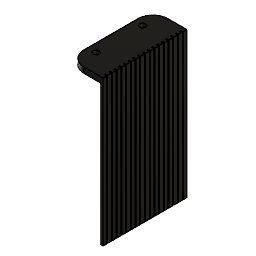
Cortina Lamas TPU (Autodesk Fusion 360 design; units mm, degrees)
Autodesk Fusion 360 part; units mm, degrees
note: some values were not read from the file. Set by a fixed rule: which sketch regions a step uses.
sketch "Boceto1" plane through (0, 0, 0) normal (0, 0, 1) x (1, 0, 0)
  circle A0 centre (0, 0) radius 1.575
  line L0 (0, 0) -> (12.5, 0)
  line L1 (12.5, 0) -> (12.5, 10)
  line L2 (12.5, 0) -> (12.5, -25)
  line L3 (12.5, 10) -> (-4.5, 10)
  line L4 (-4.5, 10) -> (-4.5, -35)
  line L5 (-4.5, -35) -> (12.5, -35)
  line L6 (12.5, -35) -> (12.5, 10)
  line L7 (12.5, -25) -> (0, -25)
  circle A1 centre (0, -25) radius 1.575
  line L8 (12.5, 10) -> (13.7, 10)
  line L9 (13.7, 10) -> (13.7, 8)
  line L10 (13.7, 8) -> (12.5, 8)
  line L11 (12.5, 8) -> (12.5, 10)
  line L12 (13.7, 5.4706) -> (12.5, 5.4706)
  line L13 (13.7, 7.4706) -> (13.7, 5.4706)
  line L14 (12.5, 7.4706) -> (13.7, 7.4706)
  line L15 (12.5, 5.4706) -> (12.5, 7.4706)
  line L16 (13.7, 2.9412) -> (12.5, 2.9412)
  line L17 (13.7, 4.9412) -> (13.7, 2.9412)
  line L18 (12.5, 4.9412) -> (13.7, 4.9412)
  line L19 (12.5, 2.9412) -> (12.5, 4.9412)
  line L20 (13.7, 0.4118) -> (12.5, 0.4118)
  line L21 (13.7, 2.4118) -> (13.7, 0.4118)
  line L22 (12.5, 2.4118) -> (13.7, 2.4118)
  line L23 (12.5, 0.4118) -> (12.5, 2.4118)
  line L24 (13.7, -2.1176) -> (12.5, -2.1176)
  line L25 (13.7, -0.1176) -> (13.7, -2.1176)
  line L26 (12.5, -0.1176) -> (13.7, -0.1176)
  line L27 (12.5, -2.1176) -> (12.5, -0.1176)
  line L28 (13.7, -4.6471) -> (12.5, -4.6471)
  line L29 (13.7, -2.6471) -> (13.7, -4.6471)
  line L30 (12.5, -2.6471) -> (13.7, -2.6471)
  line L31 (12.5, -4.6471) -> (12.5, -2.6471)
  line L32 (13.7, -7.1765) -> (12.5, -7.1765)
  line L33 (13.7, -5.1765) -> (13.7, -7.1765)
  line L34 (12.5, -5.1765) -> (13.7, -5.1765)
  line L35 (12.5, -7.1765) -> (12.5, -5.1765)
  line L36 (13.7, -9.7059) -> (12.5, -9.7059)
  line L37 (13.7, -7.7059) -> (13.7, -9.7059)
  line L38 (12.5, -7.7059) -> (13.7, -7.7059)
  line L39 (12.5, -9.7059) -> (12.5, -7.7059)
  line L40 (13.7, -12.2353) -> (12.5, -12.2353)
  line L41 (13.7, -10.2353) -> (13.7, -12.2353)
  line L42 (12.5, -10.2353) -> (13.7, -10.2353)
  line L43 (12.5, -12.2353) -> (12.5, -10.2353)
  line L44 (13.7, -14.7647) -> (12.5, -14.7647)
  line L45 (13.7, -12.7647) -> (13.7, -14.7647)
  line L46 (12.5, -12.7647) -> (13.7, -12.7647)
  line L47 (12.5, -14.7647) -> (12.5, -12.7647)
  line L48 (13.7, -17.2941) -> (12.5, -17.2941)
  line L49 (13.7, -15.2941) -> (13.7, -17.2941)
  line L50 (12.5, -15.2941) -> (13.7, -15.2941)
  line L51 (12.5, -17.2941) -> (12.5, -15.2941)
  line L52 (13.7, -19.8235) -> (12.5, -19.8235)
  line L53 (13.7, -17.8235) -> (13.7, -19.8235)
  line L54 (12.5, -17.8235) -> (13.7, -17.8235)
  line L55 (12.5, -19.8235) -> (12.5, -17.8235)
  line L56 (13.7, -22.3529) -> (12.5, -22.3529)
  line L57 (13.7, -20.3529) -> (13.7, -22.3529)
  line L58 (12.5, -20.3529) -> (13.7, -20.3529)
  line L59 (12.5, -22.3529) -> (12.5, -20.3529)
  line L60 (13.7, -24.8824) -> (12.5, -24.8824)
  line L61 (13.7, -22.8824) -> (13.7, -24.8824)
  line L62 (12.5, -22.8824) -> (13.7, -22.8824)
  line L63 (12.5, -24.8824) -> (12.5, -22.8824)
  line L64 (13.7, -27.4118) -> (12.5, -27.4118)
  line L65 (13.7, -25.4118) -> (13.7, -27.4118)
  line L66 (12.5, -25.4118) -> (13.7, -25.4118)
  line L67 (12.5, -27.4118) -> (12.5, -25.4118)
  line L68 (13.7, -29.9412) -> (12.5, -29.9412)
  line L69 (13.7, -27.9412) -> (13.7, -29.9412)
  line L70 (12.5, -27.9412) -> (13.7, -27.9412)
  line L71 (12.5, -29.9412) -> (12.5, -27.9412)
  line L72 (13.7, -32.4706) -> (12.5, -32.4706)
  line L73 (13.7, -30.4706) -> (13.7, -32.4706)
  line L74 (12.5, -30.4706) -> (13.7, -30.4706)
  line L75 (12.5, -32.4706) -> (12.5, -30.4706)
  line L76 (13.7, -35) -> (12.5, -35)
  line L77 (13.7, -33) -> (13.7, -35)
  line L78 (12.5, -33) -> (13.7, -33)
  line L79 (12.5, -35) -> (12.5, -33)
  dimension "d1" = 3.15
  dimension "d2" = 12.5
  dimension "d3" = 10
  dimension "d4" = 25
  dimension "d5" = 17
  dimension "d6" = 45
  dimension "d7" = 12.5
  dimension "d8" = 3.15
  dimension "d9" = 1.2
  dimension "d10" = 2
  dimension "d13" = 0
  dimension "d14" = -43
  constraint coincident A0.centre L0.start
  constraint horizontal L0
  constraint perpendicular L0 L1
  constraint perpendicular L0 L2
  constraint horizontal L3
  constraint vertical L4
  constraint horizontal L5
  constraint vertical L6
  constraint perpendicular L6 L7
  constraint coincident L7.end A1.centre
  constraint horizontal L8
  constraint vertical L9
  constraint horizontal L10
  constraint vertical L11
  measures "d1" diameter of A0
  measures "d2" distance of A0.centre L0.end
  measures "d3" distance of L0.end L1.end
  measures "d4" distance of L0.end L2.end
  measures "d5" distance of L1.end L3.end
  measures "d6" distance of L1.end L5.end
  measures "d7" distance of L2.end L7.end
  measures "d8" diameter of A1
  measures "d9" distance of L1.end L8.end
  measures "d10" distance of L1.end L10.end
extrude "Extruir1" add sketch "Boceto1" along normal blind 3 makes body 1
copy_body "Cuerpo - > Comp.1" bodies 1 removing the originals makes body 2 in component "Cortina de Lamas"
extrude "Extruir1'" add sketch "Boceto1" against normal blind 75 contours L1 L6 L20 L21 L22 L23 | L2 L6 L24 L25 L26 L27 | L1 L6 L16 L17 L18 L19 | L2 L6 L28 L29 L30 L31 | L1 L6 L12 L13 L14 L15 | L2 L6 L32 L33 L34 L35 | L1 L6 L8 L9 L10 L11 | L2 L6 L36 L37 L38 L39 | L2 L6 L40 L41 L42 L43 | L6 L76 L77 L78 L79 | L2 L6 L44 L45 L46 L47 | L6 L72 L73 L74 L75 | L2 L6 L48 L49 L50 L51 | L6 L68 L69 L70 L71 | L2 L6 L52 L53 L54 L55 | L6 L64 L65 L66 L67 | L2 L6 L56 L57 L58 L59 | L2 L6 L60 L61 L62 L63 bodies 2 in component "Cortina de Lamas"
fillet "Empalme1" radius 8 2 edges at (-4.5, 10, 1.5) (-4.5, -35, 1.5) on bodies 2 in component "Cortina de Lamas"
component "Cortina de Lamas" placed x (1, 0, 0) y (0, 1, 0) z (0, 0, 1) at (0, 0, 0)
named bodies: "Cortina de Lamas"
